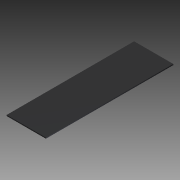
# Autodesk Inventor part: phone_cushion
Saved by Autodesk Inventor 2015 (Build 190159000, 159)
## iProperties
Created: 2015-12-01
Part Number: phone_cushion
Material: Generic
Document SubType Name: Modeling
Designer: jufranz
Density: 1 g/cm^3
Appearance: Rubber - Black
Author: jufranz
Autodesk Inventor part; units mm, degrees
ref_plane "YZ Plane" through (0, 0, 0) normal (1, 0, 0) x (0, 1, 0)
ref_plane "XZ Plane" through (0, 0, 0) normal (0, 1, 0) x (-1, 0, 0)
ref_plane "XY Plane" through (0, 0, 0) normal (0, 0, 1) x (1, 0, 0)
sketch "Sketch1" plane through (0, 0, 0) normal (0, 1, 0) x (-1, 0, 0)
  line L0 (20, 65) -> (-20, 65)
  line L1 (-20, 65) -> (-20, -65)
  line L2 (-20, -65) -> (20, -65)
  line L3 (20, -65) -> (20, 65)
  point P0 (0, 0)
  point P1 (20, 0)
  point P2 (0, 65)
  dimension "d0" = 40
  dimension "d1" = 130
  constraints: 8 end point, 2 midpoint, 2 parallel, 1 horizontal, 1 horizontal alignment, 1 perpendicular, 1 vertical alignment
  measures "d0" distance of L0.start L0.end
  measures "d1" distance of L2.end L0.start
extrude "Extrusion1" add sketch "Sketch1" along normal blind 1
body "Solid1"
